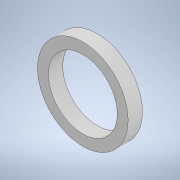
# Autodesk Inventor part: MainBoltSpacer
Saved by Autodesk Inventor 2020 (Build 240168000, 168)
## iProperties
Created: 2019-04-28
Part Number: MainBoltSpacer
Material: Generic
Document SubType Name: Modeling
Designer: Connor
Density: 1 g/cm^3
Appearance: Default
Author: Connor
Autodesk Inventor part; units mm, degrees
ref_plane "YZ Plane" through (0, 0, 0) normal (1, 0, 0) x (0, 1, 0)
ref_plane "XZ Plane" through (0, 0, 0) normal (0, 1, 0) x (-1, 0, 0)
ref_plane "XY Plane" through (0, 0, 0) normal (0, 0, 1) x (1, 0, 0)
sketch "Sketch1" plane through (0, 0, 0) normal (0, 0, 1) x (1, 0, 0)
  circle A0 centre (0, 0) radius 3.81
  circle A1 centre (0, 0) radius 5.01
  dimension "d0" = 7.62
  dimension "d1" = 1.2
  constraints: 2 centre point, 1 coincident
  measures "d0" diameter of A0
  measures "d1" radial gap between concentric circles of A0 A1
extrude "Extrusion1" add sketch "Sketch1" along normal blind 1.5875
body "Solid1"
